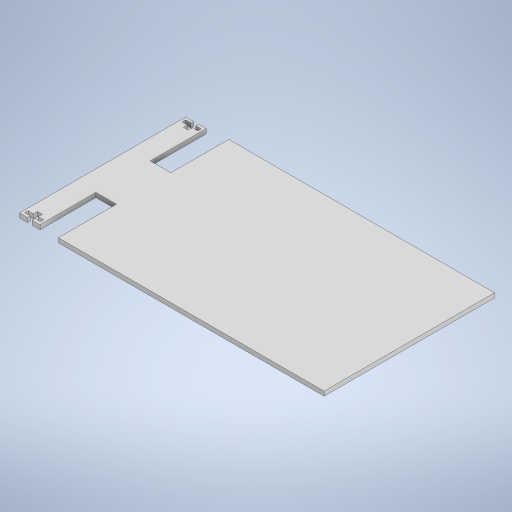
# Autodesk Inventor part: suelo_imp
Saved by Autodesk Inventor 2024 (Build 280153000, 153)
## iProperties
Created: 2023-05-01
Part Number: suelo_imp
Material: Generic
Document SubType Name: Modeling
Designer: Diego
Density: 1 g/cm^3
Appearance: Default
Author: Diego
Autodesk Inventor part; units mm, degrees
ref_plane "YZ Plane" through (0, 0, 0) normal (1, 0, 0) x (0, 1, 0)
ref_plane "XZ Plane" through (0, 0, 0) normal (0, 1, 0) x (-1, 0, 0)
ref_plane "XY Plane" through (0, 0, 0) normal (0, 0, 1) x (1, 0, 0)
sketch "Sketch1" plane through (0, 0, 0) normal (0, 1, 0) x (-1, 0, 0)
  line L0 (-97.5, -62.5) -> (97.5, -62.5)
  line L1 (97.5, 62.5) -> (-97.5, 62.5)
  line L2 (-97.5, 62.5) -> (-97.5, -62.5)
  line L3 (-97.5, -62.5) -> (97.5, 62.5) construction
  line L4 (97.5, -62.5) -> (-97.5, 62.5) construction
  line L5 (97.5, 20) -> (112.5, 20)
  line L6 (127.5, 20) -> (127.5, -20)
  line L7 (112.5, -20) -> (97.5, -20)
  line L8 (97.5, -62.5) -> (97.5, -20)
  line L9 (97.5, 20) -> (97.5, 62.5)
  line L10 (112.5, 20) -> (112.5, 61)
  line L11 (127.5, 61) -> (127.5, 20)
  line L12 (127.5, 0) -> (97.5, 0) construction
  line L13 (112.5, -20) -> (112.5, -61)
  line L14 (127.5, -61) -> (127.5, -20)
  line L15 (120, 61) -> (121.75, 61) construction
  line L16 (121.75, 61) -> (121.75, 59)
  line L17 (118.25, 61) -> (118.25, 59)
  line L18 (121.75, 59) -> (125.75, 59)
  line L19 (125.75, 59) -> (125.75, 56.5)
  line L20 (125.75, 56.5) -> (121.75, 56.5)
  line L21 (121.75, 61) -> (121.75, 53) construction
  line L22 (121.75, 56.5) -> (121.75, 53.5)
  line L23 (120, 61) -> (120, 52.3078) construction
  line L24 (118.25, 59) -> (114.25, 59)
  line L25 (114.25, 59) -> (114.25, 56.5)
  line L26 (114.25, 56.5) -> (118.25, 56.5)
  line L27 (118.25, 56.5) -> (118.25, 53.5)
  line L28 (121.75, 53.5) -> (118.25, 53.5)
  line L29 (112.5, 61) -> (118.25, 61)
  line L30 (127.5, 61) -> (121.75, 61)
  line L31 (120, -61) -> (121.75, -61) construction
  line L32 (121.75, -61) -> (121.75, -59)
  line L33 (118.25, -61) -> (118.25, -59)
  line L34 (121.75, -59) -> (125.75, -59)
  line L35 (125.75, -59) -> (125.75, -56.5)
  line L36 (125.75, -56.5) -> (121.75, -56.5)
  line L37 (121.75, -61) -> (121.75, -53) construction
  line L38 (121.75, -56.5) -> (121.75, -53.5)
  line L39 (120, -61) -> (120, -52.3078) construction
  line L40 (114.25, -56.5) -> (118.25, -56.5)
  line L41 (114.25, -59) -> (114.25, -56.5)
  line L42 (118.25, -59) -> (114.25, -59)
  line L43 (118.25, -56.5) -> (118.25, -53.5)
  line L44 (121.75, -53.5) -> (118.25, -53.5)
  line L45 (112.5, -61) -> (118.25, -61)
  line L46 (127.5, -61) -> (121.75, -61)
  point P0 (0, 0)
  dimension "d0" = 195
  dimension "d1" = 125
  dimension "d3" = 30
  dimension "d4" = 40
  dimension "d5" = 15
  dimension "d6" = 41
  dimension "d11" = 7.5
  dimension "d12" = 1.75
  dimension "d13" = 1.75
  dimension "d14" = 2
  dimension "d15" = 2
  dimension "d17" = 2.5
  dimension "d18" = 8
  dimension "d19" = 3
  dimension "d21" = 30
  dimension "d22" = 8.6922
  dimension "d23" = 1.5
  dimension "d25" = 4
  dimension "d26" = 13.25
  constraints: 94 end point, 22 symmetric about line, 11 perpendicular, 6 horizontal, 6 parallel, 3 midpoint, 3 vertical, 2 point on line
  measures "d0" distance of L1.end L1.start
  measures "d1" distance of L1.start L0.end
  measures "d3" distance of L5.start L6.start
  measures "d4" distance of L6.start L6.end
  measures "d5" distance of L5.end L6.start
  measures "d6" distance of L5.end L10.end
  measures "d11" distance of L11.start L15.start
  measures "d12" distance of L15.end L15.start
  measures "d13" distance of L15.start L17.start
  measures "d14" distance of L15.end L16.end
  measures "d15" distance of L17.start L17.end
  measures "d17" distance of L18.end L19.end
  measures "d18" distance of L15.end L21.end
  measures "d19" distance of L20.end L22.end
  measures "d21" distance from line of L12.end L11
  measures "d22" distance from line of L23.end L30
  measures "d23" distance between parallel lines of L30 L1
  measures "d25" distance of L16.end L18.end
  measures "d26" distance from line of L10.end L19
extrude "Extrusion1" add sketch "Sketch1" along normal blind 3.25
body "Solid1"
